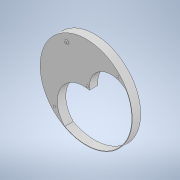
# Autodesk Inventor part: Candran face cache
Saved by Autodesk Inventor 2021 (Build 250183000, 183)
## iProperties
Created: 2020-09-18
Part Number: Candran face cache
Material: Générique
Document SubType Name: Modeling
Designer: Utilisateur
Density: 1 g/cm^3
Appearance: Par défaut
Author: Utilisateur
Autodesk Inventor part; units mm, degrees
ref_plane "YZ Plane" through (0, 0, 0) normal (1, 0, 0) x (0, 1, 0)
ref_plane "XZ Plane" through (0, 0, 0) normal (0, 1, 0) x (-1, 0, 0)
ref_plane "XY Plane" through (0, 0, 0) normal (0, 0, 1) x (1, 0, 0)
sketch "Esquisse1" plane through (0, 0, 0) normal (0, 0, 1) x (1, 0, 0)
  circle A0 centre (0, 0) radius 27
  circle A1 centre (-1.666702, -13.02482) radius 15.430073
  circle A2 centre (14.698986, 3.590179) radius 12.859707
  circle A3 centre (0, 0) radius 27.25
  circle A4 centre (0.777883, 3.425174) radius 0.684809
  circle A5 centre (-18.340493, -16.491398) radius 0.684809
  circle A6 centre (-11.511215, 19.899288) radius 1.369619
  circle A7 centre (18.687299, 17.311193) radius 0.684809
  point P0 (1.940785, 1.977619)
  point P1 (23.885419, 12.589152)
  point P2 (-12.669004, -23.843161)
  dimension "d0" = 54
  dimension "d6" = 54.5
  dimension "d9" = 1.36962
  constraints: 8 centre point, 2 coincident, 2 equal radius
  measures "d0" diameter of A0
  measures "d6" diameter of A3
  measures "d9" diameter of A4
sketch "Esquisse1 outline for Cadran" plane through (0, 0, 0) normal (0, 0, 1) x (1, 0, 0)
  circle A0 centre (0, 0) radius 27.25
  arc A1 (23.885419, 12.589152) -> (-12.669004, -23.843161) centre (0, 0) cw
  arc A2 (1.940785, 1.977619) -> (23.885419, 12.589152) centre (14.698986, 3.590179) cw
  arc A3 (-12.669004, -23.843161) -> (1.940785, 1.977619) centre (-1.666702, -13.02482) cw
extrude "Cadran" add sketch "Esquisse1 outline for Cadran" along normal blind 5
sketch "Esquisse4" plane through (0, 0, 5) normal (0, 0, 1) x (1, 0, 0)
  circle A0 centre (-11.643189, 19.963438) radius 1.192314
  circle A1 centre (0.805137, 3.454442) radius 0.685
  circle A2 centre (-18.727601, -16.711919) radius 0.685
  circle A3 centre (18.709962, 17.292624) radius 0.685
  point P0 (0, 0)
  dimension "d10" = 1.37
  constraints: 4 centre point, 2 equal radius
  measures "d10" diameter of A1
extrude "Emplacements Vis" add sketch "Esquisse4" along normal blind 0.5
fillet "Congé1" radius 0.5 1 edges at (18.025, 17.2926, 5.5)
fillet "Congé2" radius 0.5 1 edges at (0.1201, 3.4544, 5.5)
fillet "Congé3" radius 0.5 1 edges at (-12.8355, 19.9634, 5.5)
fillet "Congé4" radius 0.5 1 edges at (-19.4126, -16.7119, 5.5)
